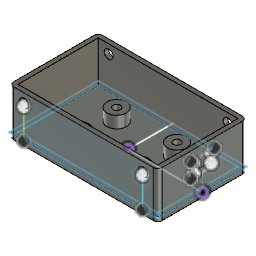
VEML7700 holder (Autodesk Fusion 360 design; units mm, degrees)
part number: 2026-05-14-21-16-27-121
Autodesk Fusion 360 part; units mm, degrees
sketch "sensor holes" plane through (0, 0, 0) normal (0, 0, 1) x (1, 0, 0)
  line L0 (-10.16, 6.35) -> (10.16, 6.35) construction
  line L1 (10.16, 6.35) -> (10.16, -6.35) construction
  line L2 (10.16, -6.35) -> (-10.16, -6.35) construction
  line L3 (-10.16, -6.35) -> (-10.16, 6.35) construction
  line L4 (0, 6.35) -> (0, -6.35) construction
  circle A0 centre (-10.16, 6.35) radius 1.25
  circle A1 centre (10.16, 6.35) radius 1.25
  line L5 (0, 6.35) -> (0, -6.35) construction
  line L6 (-10.16, 0) -> (10.16, 0) construction
  circle A2 centre (-10.16, -6.35) radius 1.25
  circle A3 centre (10.16, -6.35) radius 1.25
  point P0 (0, 6.35)
  point P1 (0, -6.35)
  dimension "d1" = 20.32
  dimension "d2" = 12.7
  dimension "d3" = 2.5
  constraint horizontal L0
  constraint perpendicular L0 L1
  constraint perpendicular L1 L2
  constraint perpendicular L0 L3
  constraint midpoint L0 P0
  constraint midpoint L2 P1
  constraint coincident P0 L4.start
  constraint coincident P1 L4.end
  constraint midpoint L4 origin
  constraint coincident L0.start L3.end
  constraint symmetric P0 L4 L5.start
  constraint symmetric P1 L4 L5.end
  constraint symmetric L4 A0 A1
  constraint midpoint L3 L6.start
  constraint midpoint L1 L6.end
  constraint symmetric A0 L6 A2
  constraint symmetric A1 L6 A3
  measures "d1" distance of L0.start L0.end
  measures "d2" distance of L0.end L1.end
  measures "d3" diameter of A0
extrude "Extrude1" add sketch "sensor holes" along normal blind 4 thin wall 2 outside makes body 1 at (-6.914, 6.188, 2.6667) makes body 2 at (13.406, 6.188, 2.6667) makes body 3 at (-6.914, -6.512, 2.6667) makes body 4 at (13.406, -6.512, 2.6667)
sketch "bottom" plane through (0, 0, 0) normal (0, 0, 1) x (1, 0, 0)
  line L0 (-25, 15) -> (25, 15)
  line L1 (25, 15) -> (25, -15)
  line L2 (25, -15) -> (-25, -15)
  line L3 (-25, -15) -> (-25, 15)
  line L4 (0, 15) -> (0, 0)
  line L5 (25, 0) -> (0, 0)
  line L6 (-23.5, 13.5) -> (23.5, 13.5)
  line L7 (23.5, 13.5) -> (23.5, -13.5)
  line L8 (23.5, -13.5) -> (-23.5, -13.5)
  line L9 (-23.5, -13.5) -> (-23.5, 13.5)
  dimension "d7" = 1.5
  constraint horizontal L0
  constraint vertical L1
  constraint horizontal L2
  constraint vertical L3
  constraint midpoint L0 L4.start
  constraint coincident L4.end L5.end
  constraint perpendicular L0 L4
  constraint midpoint L1 L5.start
  constraint perpendicular L4 L5
extrude "Extrude2" add sketch "bottom" against normal blind 1.5 bodies 1 2 3 4
extrude "Extrude3" add sketch "bottom" along normal blind 14 separate body contours L0 L1 L2 L3 L4 L5 L6 L7 L8 L9 | L0 L1 L4 L5 L6 L7 makes body 5
fillet "Fillet1" radius 1.5 1 edges at (25, -15, 7) on bodies 5
fillet "Fillet2" radius 1.5 1 edges at (25, 15, 7) on bodies 5
fillet "Fillet3" radius 1.5 1 edges at (-25, -15, 7) on bodies 5
fillet "Fillet4" radius 1.5 1 edges at (-25, 15, 7) on bodies 5
fillet "Fillet5" radius 1.5 1 edges at (-25, 15, -0.75) on bodies 1
fillet "Fillet6" radius 1.5 1 edges at (-25, -15, -0.75) on bodies 1
fillet "Fillet7" radius 1.5 1 edges at (25, -15, -0.75) on bodies 1
fillet "Fillet8" radius 1.5 1 edges at (25, 15, -0.75) on bodies 1
sketch "side" plane through (0, -15, 0) normal (0, -1, 0) x (1, 0, 0)
  line L0 (-23.5, 14) -> (-23.5, 0)
  line L1 (-23.5, 0) -> (23.5, 0)
  line L2 (23.5, 0) -> (23.5, 14)
  line L3 (23.5, 14) -> (-23.5, 14)
  line L4 (-20, 0) -> (-20, 10)
  line L5 (20, 0) -> (20, 10)
  dimension "d43" = 10
  dimension "d44" = 10
  constraint coincident L1 L4.start
  constraint perpendicular L1 L4
  constraint coincident L1 L5.start
  constraint perpendicular L1 L5
  measures "d43" distance of L4.start L4.end
  measures "d44" distance of L5.start L5.end
hole "Hole1" at (-20, -15, 11) direction (0, 1, 0) diameter 3 depth 32 tip angle 118 bodies 5
hole "Hole2" at (20, -15, 11) direction (0, 1, 0) diameter 3 depth 32 tip angle 118 bodies 5
sketch "STEMMA" plane through (25, 0, 0) normal (1, 0, 0) x (0, 1, 0)
  line L0 (13.5, 0) -> (13.5, 14)
  line L1 (13.5, 14) -> (-13.5, 14)
  line L2 (-13.5, 14) -> (-13.5, 0)
  line L3 (-13.5, 0) -> (13.5, 0)
  line L4 (0, 0) -> (0, 6) construction
  line L5 (-3, 11) -> (3, 11)
  line L6 (4, 10) -> (4, 7)
  line L7 (3, 6) -> (-3, 6)
  line L8 (-4, 7) -> (-4, 10)
  arc A0 (-3, 11) -> (-4, 10) centre (-3, 10) ccw
  arc A1 (4, 10) -> (3, 11) centre (3, 10) ccw
  arc A2 (-4, 7) -> (-3, 6) centre (-3, 7) ccw
  arc A3 (3, 6) -> (4, 7) centre (3, 7) ccw
  point P0 (-4, 11)
  point P1 (4, 11)
  point P2 (-4, 6)
  dimension "d34" = 8
  dimension "d35" = 5
  dimension "d36" = 1
  dimension "d37" = 1
  dimension "d38" = 1
  dimension "d39" = 1
  dimension "d42" = 6
  constraint coincident L4.start origin
  constraint perpendicular L3 L4
  constraint horizontal L5
  constraint vertical L6
  constraint horizontal L7
  constraint vertical L8
  constraint coincident P0 L5
  constraint coincident P0 L8
  constraint tangent L5 A0
  constraint tangent L8 A0
  constraint coincident P1 L5
  constraint coincident P1 L6
  constraint tangent L5 A1
  constraint tangent L6 A1
  constraint coincident L4.end L7
  constraint coincident P2 L7
  constraint coincident P2 L8
  constraint tangent L7 A2
  constraint tangent L8 A2
  constraint tangent L6 A3
  constraint tangent L7 A3
  measures "d34" distance of P0 P1
  measures "d35" distance of P0 P2
  measures "d36" radius of A0
  measures "d37" radius of A1
  measures "d38" radius of A2
  measures "d39" radius of A3
  measures "d42" distance of L4.start L4.end
extrude "Extrude4" cut sketch "STEMMA" against normal blind 1.5 contours L5 L6 L7 L8 A0 A1 A2 A3 bodies 5
equation "d43 = attachHoleHeight"
equation "d44 = attachHoleHeight"
equation "attachHoleHeight = 10 mm"
